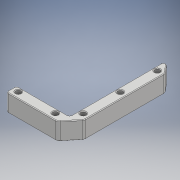
# Autodesk Inventor part: dual_motor_spacer_1
Saved by Autodesk Inventor 2018 (Build 220112000, 112)
## iProperties
Created: 2018-05-01
Part Number: dual_motor_spacer_1
Material: Generic
Document SubType Name: Modeling
Designer: mshaw2
Density: 1 g/cm^3
Appearance: Default
Author: mshaw2
## iProperties of the stored document dual_motor_spacer_1_3DPrint.ipt
Created: 2018-05-01
Part Number: dual_motor_spacer_1_3DPrint
Material: Generic
Document SubType Name: Modeling
Designer: mshaw2
Density: 1 g/cm^3
Appearance: Default
Author: mshaw2
Autodesk Inventor part; units mm, degrees
ref_plane "YZ Plane" through (0, 0, 0) normal (1, 0, 0) x (0, 1, 0)
ref_plane "XZ Plane" through (0, 0, 0) normal (0, 1, 0) x (-1, 0, 0)
ref_plane "XY Plane" through (0, 0, 0) normal (0, 0, 1) x (1, 0, 0)
sketch "Sketch1" plane through (0, 0, 0) normal (0, 0, 1) x (1, 0, 0)
  arc A0 (-0.3454, 49.9645) -> (-0.9, 48.8) centre (0.6, 48.8) ccw construction
  arc A1 (-0.3454, 49.9645) -> (-1.3157, 49.3765) centre (0, 48.3) ccw construction
  line L0 (-1.3157, 49.3765) -> (-5.8157, 43.8765) construction
  arc A2 (-5.8157, 43.8765) -> (-6.2, 42.8) centre (-4.5, 42.8) ccw construction
  line L1 (-6.2, 42.8) -> (-6.2, 7.2) construction
  arc A3 (-6.2, 7.2) -> (-5.8157, 6.1235) centre (-4.5, 7.2) ccw construction
  line L2 (-5.8157, 6.1235) -> (-1.3157, 0.6235) construction
  arc A4 (-1.3157, 0.6235) -> (0, 0) centre (0, 1.7) ccw construction
  line L3 (0, 0) -> (22.6, 0) construction
  arc A5 (22.6, 0) -> (23.9157, 0.6235) centre (22.6, 1.7) ccw construction
  line L4 (23.9157, 0.6235) -> (28.4157, 6.1235) construction
  arc A6 (28.4157, 6.1235) -> (28.8, 7.2) centre (27.1, 7.2) ccw construction
  line L5 (28.8, 7.2) -> (28.8, 42.8) construction
  arc A7 (28.8, 42.8) -> (28.4157, 43.8765) centre (27.1, 42.8) ccw construction
  line L6 (28.4157, 43.8765) -> (23.9157, 49.3765) construction
  arc A8 (23.9157, 49.3765) -> (22.9454, 49.9645) centre (22.6, 48.3) ccw construction
  arc A9 (23.5, 48.8) -> (22.9454, 49.9645) centre (22, 48.8) ccw construction
  line L7 (23.5, 48.8) -> (23.5, 6.8) construction
  arc A10 (22, 5.3) -> (23.5, 6.8) centre (22, 6.8) ccw construction
  line L8 (0.6, 5.3) -> (22, 5.3) construction
  arc A11 (-0.9, 6.8) -> (0.6, 5.3) centre (0.6, 6.8) ccw construction
  line L9 (-0.9, 48.8) -> (-0.9, 6.8) construction
  circle A12 centre (2.8, 2.5) radius 1.2
  circle A13 centre (19.8, 2.5) radius 1.2
  circle A14 centre (-3.7, 42.8) radius 1.2 construction
  circle A15 centre (-3.7, 25.8) radius 1.2 construction
  circle A16 centre (-3.7, 8.8) radius 1.2 construction
  circle A17 centre (26.3, 8.8) radius 1.2
  circle A18 centre (26.3, 25.8) radius 1.2
  circle A19 centre (26.3, 42.8) radius 1.2
  line L10 (22.6, -0.3) -> (0, -0.3) construction
  arc A20 (-1.5479, 0.4335) -> (0, -0.3) centre (0, 1.7) ccw construction
  line L11 (-1.5479, 0.4335) -> (-6.0479, 5.9335) construction
  arc A21 (-6.5, 7.2) -> (-6.0479, 5.9335) centre (-4.5, 7.2) ccw construction
  line L12 (-6.5, 7.2) -> (-6.5, 42.8) construction
  line L13 (28.6479, 5.9335) -> (24.1479, 0.4335) construction
  arc A22 (22.6, -0.3) -> (24.1479, 0.4335) centre (22.6, 1.7) ccw construction
  line L14 (29.1, 42.8) -> (29.1, 7.2) construction
  arc A23 (28.6479, 5.9335) -> (29.1, 7.2) centre (27.1, 7.2) ccw construction
  arc A24 (29.1, 42.8) -> (28.6479, 44.0665) centre (27.1, 42.8) ccw construction
  line L15 (24.1479, 49.5665) -> (28.6479, 44.0665) construction
  arc A25 (24.1479, 49.5665) -> (22.6, 50.3) centre (22.6, 48.3) ccw construction
  spline S0 degree 3 poles (22.6, 50.1748) (22.6318, 50.1609) (22.6649, 50.1451) (22.7851, 50.0818) (22.8689, 50.0267) (22.9454, 49.9645) knots -0.198467 -0.198467 -0.198467 -0.198467 -0.191756 -0.191756 -0.174636 -0.174636 -0.174636 -0.174636 construction
  spline S1 degree 3 poles (22.6, 50.1748) (22.5559, 50.194) (22.511, 50.2111) (22.3105, 50.2765) (22.1493, 50.3) (22, 50.3) knots -0.063423 -0.063423 -0.063423 -0.063423 -0.049053 -0.049053 0 0 0 0 construction
  arc A26 (0, 50.3) -> (-1.5479, 49.5665) centre (0, 48.3) ccw construction
  line L16 (0, 50.3) -> (0.6, 50.3) construction
  line L17 (-6.0479, 44.0665) -> (-1.5479, 49.5665) construction
  spline S2 degree 3 poles (0, 50.1748) (-0.0932, 50.1341) (-0.1972, 50.077) (-0.3151, 49.9887) (-0.3305, 49.9767) (-0.3454, 49.9645) knots 0.037429 0.037429 0.037429 0.037429 0.058499 0.058499 0.061766 0.061766 0.061766 0.061766 construction
  spline S3 degree 3 poles (0.6, 50.3) (0.4507, 50.3) (0.2895, 50.2765) (0.089, 50.2111) (0.0441, 50.194) (0, 50.1748) knots -0.307639 -0.307639 -0.307639 -0.307639 -0.258586 -0.258586 -0.244216 -0.244216 -0.244216 -0.244216 construction
  line L18 (22, 50.3) -> (22.6, 50.3) construction
  arc A27 (-6.0479, 44.0665) -> (-6.5, 42.8) centre (-4.5, 42.8) ccw construction
  circle A28 centre (11.3, 38.3) radius 5 construction
  line L19 (24.3, 49.3806) -> (24.3, 4.5)
  line L20 (24.3, 49.3806) -> (28.6479, 44.0665)
  line L21 (29.1, 42.8) -> (29.1, 7.2)
  line L22 (28.6479, 5.9335) -> (24.1479, 0.4335)
  line L23 (22.6, -0.3) -> (0, -0.3)
  line L24 (0, -0.3) -> (0, 4.5)
  line L25 (24.3, 4.5) -> (0, 4.5)
  arc A29 (28.6479, 5.9335) -> (29.1, 7.2) centre (27.1, 7.2) ccw
  arc A30 (22.6, -0.3) -> (24.1479, 0.4335) centre (22.6, 1.7) ccw
  arc A31 (29.1, 42.8) -> (28.6479, 44.0665) centre (27.1, 42.8) ccw
  point P0 (11.3, 25)
  dimension "d1" = 0.8
  dimension "d2" = 0.8
  constraints: 52 end point, 46 point on circle, 32 centre point, 7 vertical, 5 horizontal, 3 coincident, 3 collinear, 2 perpendicular, 1 parallel, 1 point on line, 122 other
  measures "d1" distance between parallel lines of L7 L19
  measures "d2" distance between parallel lines of L25 L8
extrude "Extrusion1" add sketch "Sketch1" along normal blind 8
fillet "Fillet1" radius 1 4 edges at (24.3, 4.5, 4) (24.3, 49.3806, 4) (0, 4.5, 4) (0, -0.3, 4)
fillet "Fillet1" radius 0.3 30 edges at (25.1, 42.8, 8) (25.1, 25.8, 8) (25.1, 8.8, 8) (18.6, 2.5, 8) (1.6, 2.5, 8) (25.1, 8.8, 0) (25.1, 25.8, 0) (25.1, 42.8, 0) (18.6, 2.5, 0) (1.6, 2.5, 0) (23.4565, -0.1073, 0) (11.3, -0.3, 0) (28.9836, 6.5276, 0) (29.1, 25, 0) (28.9836, 43.4724, 0) (26.474, 46.7235, 0) (26.3979, 3.1835, 0) (24.3, 26.9403, 0) (12.15, 4.5, 0) (0, 2.1, 0) (0, 2.1, 8) (23.4565, -0.1073, 8) (26.3979, 3.1835, 8) (28.9836, 6.5276, 8) (29.1, 25, 8) (28.9836, 43.4724, 8) (26.474, 46.7235, 8) (11.3, -0.3, 8) (12.15, 4.5, 8) (24.3, 26.9403, 8)
equation "\"d2\" = d1"
equation "\"d0\" = d1"
body "Solid1"
